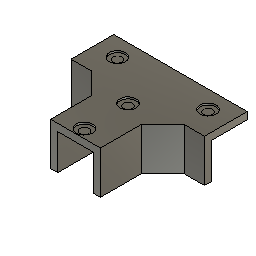
Bed Bracket V2 (Autodesk Fusion 360 design; units mm, degrees)
Autodesk Fusion 360 part; units mm, degrees
sketch "Sketch1" plane through (0, 0, 0) normal (0, 1, 0) x (1, 0, 0)
  line L0 (25, -10) -> (-50, -10)
  line L1 (-50, -10) -> (-50, 14)
  line L2 (-50, 14) -> (25, 14)
  line L3 (25, 14) -> (25, -10)
  line L4 (25, -10) -> (-50, 14) construction
  line L5 (-50, -10) -> (25, 14) construction
  point P0 (-12.5, 2)
  dimension "d1" = 75
  dimension "d2" = 24
  constraint perpendicular L0 L1
  constraint parallel L0 L2
  constraint parallel L1 L3
  constraint horizontal L0
  constraint coincident L4 P0
  constraint coincident L5 P0
  measures "d1" distance of L1.end L2.end
  measures "d2" distance of L0.end L1.end
extrude "Extrude1" add sketch "Sketch1" along normal blind 24
sketch "Sketch5" plane through (0, 0, 0) normal (0, -1, 0) x (1, 0, 0)
  line L0 (25, -14) -> (25, 10)
  line L1 (25, 10) -> (-50, 10)
  line L2 (-50, 10) -> (-50, -14)
  line L3 (1.5, 10) -> (-26.5, 10)
  line L4 (-26.5, 10) -> (-26.5, -14)
  line L5 (-26.5, -14) -> (1.5, -14)
  line L6 (1.5, -14) -> (1.5, 10)
  line L7 (1.5, 10) -> (-26.5, -14) construction
  line L8 (-26.5, 10) -> (1.5, -14) construction
  line L9 (-50, -14) -> (25, -14)
  dimension "d15" = 24
  dimension "d16" = 28
  dimension "d232" = 23.5
  constraint perpendicular L3 L4
  constraint parallel L3 L5
  constraint parallel L4 L6
  constraint horizontal L3
  measures "d15" distance of L3.end L4.end
  measures "d16" distance of L4.end L5.end
  measures "d232" distance of L0 L6
extrude "Extrude3" add sketch "Sketch5" along normal blind 35 contours L1 L3 L4 L5 L6 L9
sketch "Sketch6" plane through (0, -35, 0) normal (0, -1, 0) x (1, 0, 0)
  line L0 (1.5, -14) -> (1.5, 10)
  line L1 (1.5, 10) -> (-26.5, 10)
  line L2 (-26.5, 10) -> (-26.5, -14)
  line L3 (-26.5, -14) -> (1.5, -14)
  line L4 (-2.5, 6) -> (-22.5, 6)
  line L5 (-22.5, 6) -> (-22.5, -14)
  line L6 (-22.5, -14) -> (-2.5, -14)
  line L7 (-2.5, -14) -> (-2.5, 6)
  line L8 (-2.5, 6) -> (-22.5, -14) construction
  line L9 (-22.5, 6) -> (-2.5, -14) construction
  line L10 (-12.5, -2) -> (-12.5, -4) construction
  point P0 (-12.5, -4)
  dimension "d19" = 20
  dimension "d20" = 20
  dimension "d46" = 2
  dimension "d233" = 4
  constraint perpendicular L4 L5
  constraint parallel L4 L6
  constraint parallel L5 L7
  constraint horizontal L4
  constraint coincident L8 P0
  constraint coincident L9 P0
  constraint parallel L5 L10
  constraint coincident P0 L10.end
  measures "d19" distance of L4.end L5.end
  measures "d20" distance of L5.end L6.end
  measures "d46" distance of L10.start P0
  measures "d233" distance of L2 L5
extrude "Extrude4" cut sketch "Sketch6" against normal blind 44 contours L3 L4 L5 L6 L7
sketch "Sketch14" plane through (-50, 0, 0) normal (-1, 0, 0) x (0, -1, 0)
  line L0 (0, -14) -> (0, 10)
  line L1 (0, 10) -> (-24, 10)
  line L2 (-24, 10) -> (-24, -14)
  line L3 (-24, -14) -> (0, -14)
  line L4 (-20, -14) -> (-20, 10) construction
  line L5 (-4, 10) -> (-4, -14) construction
  line L6 (-4, -14) -> (-24, -14)
  line L7 (-24, -14) -> (-24, 6)
  line L8 (-24, 6) -> (-4, 6)
  line L9 (-4, 6) -> (-4, -14)
  dimension "d112" = 4
  dimension "d113" = 4
  dimension "d114" = 20
  constraint coincident L3 L4.start
  constraint coincident L1 L4.end
  constraint perpendicular L1 L4
  constraint coincident L1 L5.start
  constraint coincident L3 L5.end
  constraint perpendicular L3 L5
  constraint horizontal L6
  constraint vertical L7
  constraint horizontal L8
  constraint vertical L9
  measures "d112" distance of L0 L5
  measures "d113" distance of L2 L4
  measures "d114" distance of L5.end L8.end
extrude "Extrude22" cut sketch "Sketch14" against normal blind 100 contours L2 L3 L6 L7 L8 L9
sketch "Sketch18" plane through (0, 0, 10) normal (0, 0, 1) x (-1, 0, 0)
  line L0 (-1.5, 0) -> (-25, 0)
  line L1 (-25, 0) -> (-25, -24)
  line L2 (-25, -24) -> (50, -24)
  line L3 (50, -24) -> (50, 0)
  circle A0 centre (-13, -14) radius 4.5
  circle A1 centre (38, -14) radius 4.5
  circle A2 centre (12.5, 5.5) radius 4.5
  circle A3 centre (12.5, 30) radius 4.5
  line L4 (26.5, 0) -> (26.5, 35)
  line L5 (26.5, 35) -> (-1.5, 35)
  line L6 (-1.5, 35) -> (-1.5, 0)
  line L7 (50, 0) -> (26.5, 0)
  circle A4 centre (38, -14) radius 2.5
  circle A5 centre (12.5, 5.5) radius 2.5
  circle A6 centre (12.5, 30) radius 2.5
  circle A7 centre (-13, -14) radius 2.5
  line L8 (12.5, 35) -> (12.5, -24) construction
  line L9 (-25, -14) -> (50, -14) construction
  line L10 (-1.5, 25) -> (26.5, 25) construction
  dimension "d70" = 9
  dimension "d72" = 9
  dimension "d73" = 9
  dimension "d74" = 9
  dimension "d219" = 5
  dimension "d220" = 5
  dimension "d221" = 5
  dimension "d222" = 5
  dimension "d235" = 10
  dimension "d236" = 12
  dimension "d237" = 12
  dimension "d238" = 10
  constraint concentric A1 A4
  constraint concentric A2 A5
  constraint concentric A3 A6
  constraint concentric A0 A7
  constraint midpoint L5 L8.start
  constraint midpoint L2 L8.end
  constraint coincident L1 L9.start
  constraint coincident L3 L9.end
  constraint perpendicular L3 L9
  constraint coincident A0.centre L9
  constraint coincident A3.centre L8
  constraint midpoint A2.centre L8
  constraint coincident L6 L10.start
  constraint coincident L4 L10.end
  constraint perpendicular L4 L10
  measures "d70" diameter of A0
  measures "d72" diameter of A1
  measures "d73" diameter of A2
  measures "d74" diameter of A3
  measures "d219" diameter of A4
  measures "d220" diameter of A5
  measures "d221" diameter of A6
  measures "d222" diameter of A7
  measures "d235" distance of L2 L9
  measures "d236" distance of L3 A1.centre
  measures "d237" distance of L1 A0.centre
  measures "d238" distance of L5 L10
extrude "Extrude44" cut sketch "Sketch18" against normal up to surface (2.8 mm away) from surface at -1.2 contours A4 | A5 | A6 | A7
extrude "Extrude15" cut sketch "Sketch18" against normal blind 1 contours A0 | A1 | A2 | A3 | A4 | A5 | A6 | A7
chamfer "Chamfer12" distance 12 angle 45 2 edges at (-26.5, 0, -2) (1.5, 0, -2)
